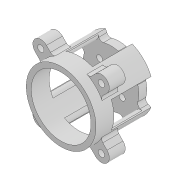
# Autodesk Inventor part: Motor Mount
Saved by Autodesk Inventor 2020 (Build 240168000, 168)
## iProperties
Created: 2020-04-09
Part Number: Motor Mount
Material: Generic
Document SubType Name: Modeling
Designer: John K
Density: 1 g/cm^3
Appearance: Default
Author: John K
Autodesk Inventor part; units mm, degrees
ref_plane "YZ Plane" through (0, 0, 0) normal (1, 0, 0) x (0, 1, 0)
ref_plane "XZ Plane" through (0, 0, 0) normal (0, 1, 0) x (-1, 0, 0)
ref_plane "XY Plane" through (0, 0, 0) normal (0, 0, 1) x (1, 0, 0)
sketch "Sketch1" plane through (0, 0, 0) normal (0, 0, 1) x (1, 0, 0)
  circle A0 centre (0, 0) radius 17.5
  dimension "d0" = 35
  constraints: 1 centre point, 1 coincident
  measures "d0" diameter of A0
extrude "Extrusion1" add sketch "Sketch1" along normal blind 4
sketch "Sketch2" plane through (0, 0, 4) normal (0, 0, 1) x (1, 0, 0)
  circle A0 centre (0, 0) radius 17.5 projected
  circle A1 centre (0, 0) radius 15
  dimension "d3" = 2.5
  constraints: 1 centre point
  measures "d3" radial gap between concentric circles of A0 A1
extrude "Length" add sketch "Sketch2" along normal blind 25
sketch "Sketch3" plane through (0, 0, 0) normal (0, 0, -1) x (-1, 0, 0)
  circle A0 centre (0, 0) radius 17.5 projected
  line L0 (0, 0) -> (-12.9343, 5.3576)
  line L1 (0, 0) -> (-12.9343, -5.3576)
  line L2 (0, 0) -> (-17.5, 0) construction
  line L3 (-12.9343, 5.3576) -> (-16.1679, 6.697)
  line L4 (-12.9343, -5.3576) -> (-16.1679, -6.697)
  arc A1 (-12.9343, 5.3576) -> (-12.9343, -5.3576) centre (0, 0) ccw
  dimension "d6" = 45
  dimension "d7" = 22.5
  dimension "d10" = 14
  constraints: 10 end point, 5 point on circle, 2 collinear, 1 centre point, 1 coincident, 1 horizontal
  measures "d6" angle of L0 L1
  measures "d7" angle of L0 L2
  measures "d10" radius of A1
extrude "Extrusion3" cut sketch "Sketch3" against normal blind 20 contours L3 A1 L4 A0
fillet "Fillet1" radius 2 2 edges at (12.9343, 5.3576, 2) (12.9343, -5.3576, 2)
fillet "Fillet2" radius 2 2 edges at (13.9342, 5.5531, 12) (13.9342, -5.5531, 12)
pattern_circular "Circular Pattern1" count 4 over 360 about axis through (0, 0, 0) along (0, 0, 1) of "Fillet2", "Fillet1", "Extrusion3"
sketch "Sketch4" plane through (0, 0, 0) normal (0, 0, -1) x (-1, 0, 0)
  arc A0 (3.6988, 13.5026) -> (-3.6988, 13.5026) centre (0, 0) ccw projected
  constraints: 1 coincident
hole "Hole1" at (0, 0, 0) direction (0, 0, 1) diameter 8.2 end through all
sketch "Sketch5" plane through (0, 0, 0) normal (0, 0, -1) x (-1, 0, 0)
  line L0 (-6.7175, 6.7175) -> (6.7175, 6.7175) construction
  line L1 (6.7175, 6.7175) -> (6.7175, -6.7175) construction
  line L2 (6.7175, -6.7175) -> (-6.7175, -6.7175) construction
  line L3 (-6.7175, -6.7175) -> (-6.7175, 6.7175) construction
  line L4 (-6.7175, 6.7175) -> (6.7175, -6.7175) construction
  line L5 (6.7175, 6.7175) -> (-6.7175, -6.7175) construction
  point P0 (0, 0)
  dimension "d23" = 19
  constraints: 12 end point, 2 coincident, 2 midpoint, 2 parallel, 2 perpendicular, 1 horizontal
  measures "d23" distance of L0.start L1.end
hole "Hole2" at (6.7175, 6.7175, 0) at (-6.7175, -6.7175, 0) direction (0, 0, 1) diameter 3 end through all clearance for "Flat Head Machine Screw" size "M3" standard "Ansi Metric M Profile"
sketch "Sketch6" plane through (0, 0, 0) normal (0, 0, -1) x (-1, 0, 0)
  line L0 (-5.6569, -5.6569) -> (5.6569, -5.6569) construction
  line L1 (5.6569, -5.6569) -> (5.6569, 5.6569) construction
  line L2 (5.6569, 5.6569) -> (-5.6569, 5.6569) construction
  line L3 (-5.6569, 5.6569) -> (-5.6569, -5.6569) construction
  line L4 (-5.6569, -5.6569) -> (5.6569, 5.6569) construction
  line L5 (5.6569, -5.6569) -> (-5.6569, 5.6569) construction
  point P0 (0, 0)
  dimension "d31" = 16
  constraints: 12 end point, 2 coincident, 2 midpoint, 2 parallel, 2 perpendicular, 1 horizontal
  measures "d31" distance of L0.start L1.end
hole "Hole3" at (-5.6569, 5.6569, 0) at (5.6569, -5.6569, 0) direction (0, 0, 1) diameter 3 end through all
ref_plane "Work Plane1" through (0, 0, 24) normal (0, 0, 1) x (1, 0, 0)
sketch "Sketch7" plane through (0, 0, 24) normal (0, 0, 1) x (1, 0, 0)
  line L0 (0, 0) -> (-12.3744, 12.3744) construction
  circle A0 centre (0, 0) radius 17.5 construction
  line L1 (0, 0) -> (-17.5, 0) construction
  circle A1 centre (-15.2028, 15.2028) radius 4
  circle A2 centre (0, 0) radius 15 projected
  arc A3 (-7.3308, 13.0866) -> (-13.0866, 7.3308) centre (0, 0) ccw projected
  line L2 (-18.059, 12.4025) -> (-13.0866, 7.3308)
  line L3 (-12.3465, 18.0031) -> (-7.4565, 13.0154)
  dimension "d39" = 45
  dimension "d40" = 8
  constraints: 8 end point, 5 point on circle, 3 tangent, 1 centre point, 1 horizontal, 1 parallel, 1 point on line
  measures "d39" angle of L0 L1
  measures "d40" diameter of A1
extrude "Extrusion4" add sketch "Sketch7" against normal blind 8 contours A1 | A1 L3 A2 L2
fillet "Fillet3" radius 2 2 edges at (-14.8992, 9.1795, 20) (-9.2566, 14.8515, 20)
sketch "Sketch8" plane through (0, 0, 16) normal (0, 0, -1) x (-1, 0, 0)
  arc A0 (18.059, 12.4025) -> (12.3465, 18.0031) centre (15.2028, 15.2028) ccw projected
  point P0 (0, 0)
  constraints: 1 coincident
hole "Hole4" at (-15.2028, 15.2028, 16) direction (0, 0, 1) diameter 3.2 end through all counterbore diameter 6.5 counterbore depth 3 clearance for "Socket Head Cap Screw" size "M3" standard "Ansi Metric M Profile"
pattern_circular "Circular Pattern2" count 4 over 360 about axis through (0, 0, 0) along (0, 0, 1) of "Hole4", "Fillet3", "Extrusion4"
equation "\"d7\" = 0.5 * d6"
body "Solid1"
